C Clamp Render (Autodesk Fusion 360 archive; units mm, degrees)
design "Main Body"
part number: 2026-06-23-09-52-08-828
Autodesk Fusion 360 part; units mm, degrees
sketch "Sketch1" plane through (0, 0, 0) normal (0, 1, 0) x (1, 0, 0)
  spline S0 degree 5 poles (-77.228, -92.7344) (-75.7321, -92.7465) (-72.7402, -92.7709) (-68.2525, -92.8074) (-62.2689, -92.856) (-54.7893, -92.9168) (-48.8056, -92.9655) (-44.3179, -93.0019) (-41.3261, -93.0263) (-39.8302, -93.0384) knots 0 0 0 0 0 0 0.2 0.4 0.6 0.8 1 1 1 1 1 1
  spline S1 degree 5 poles (0, -10) (0, -14) (0, -22) (0, -34) (0, -50) (0, -70) (0, -86) (0, -98) (0, -106) (0, -110) knots 0 0 0 0 0 0 0.2 0.4 0.6 0.8 1 1 1 1 1 1
  spline S2 degree 5 poles (0, -110) (-0.2419, -110.8286) (-0.8048, -112.4078) (-1.8868, -114.5428) (-3.8082, -116.9186) (-7.0161, -119.0978) (-11.0197, -120.5038) (-15.7646, -121.2051) (-21.1395, -121.3347) (-27.004, -121.0593) (-33.2045, -120.5595) (-39.5939, -120.0074) (-46.047, -119.5474) (-52.4786, -119.2731) (-58.8364, -119.2387) (-65.0917, -119.4702) (-70.0044, -119.8743) (-73.6364, -120.2998) (-76.0347, -120.6375) (-77.228, -120.8199) knots 0 0 0 0 0 0 0.066667 0.133333 0.2 0.266667 0.333333 0.4 0.466667 0.533333 0.6 0.666667 0.733333 0.8 0.866667 0.933333 1 1 1 1 1 1
  spline S3 degree 5 poles (-39.8302, -93.0384) (-39.4353, -93.0976) (-38.6638, -93.1866) (-37.5612, -93.2318) (-36.2024, -93.1125) (-34.7008, -92.6456) (-33.4105, -91.8376) (-32.3432, -90.6698) (-31.496, -89.1468) (-30.8521, -87.2956) (-30.3924, -85.1473) (-30.158, -83.2133) (-30.0522, -81.6499) (-30.0123, -80.5582) (-30, -80) knots 0 0 0 0 0 0 0.1 0.2 0.3 0.4 0.5 0.6 0.7 0.8 0.9 1 1 1 1 1 1
  line L0 (-30, -80) -> (-30, -10)
  spline S4 degree 5 poles (-30, -10) (-30.0155, -9.1002) (-30.1233, -7.3553) (-30.5152, -4.9016) (-31.5056, -1.9629) (-33.5686, 1.1235) (-36.5062, 3.5878) (-40.343, 5.4122) (-45.0325, 6.6301) (-50.4945, 7.2984) (-56.6452, 7.4768) (-62.0611, 7.267) (-66.3821, 6.9254) (-69.376, 6.6171) (-70.9013, 6.4428) knots 0 0 0 0 0 0 0.1 0.2 0.3 0.4 0.5 0.6 0.7 0.8 0.9 1 1 1 1 1 1
  line L1 (-70.9013, 6.4428) -> (-70.9013, -3.3971)
  line L2 (-70.9013, -3.3971) -> (-100.9013, -3.3971)
  spline S5 degree 5 poles (-100.9013, -3.3971) (-100.9574, -2.1416) (-101.0166, 0.3245) (-100.9463, 3.8888) (-100.5294, 8.3669) (-99.4326, 13.476) (-97.7071, 18.0518) (-95.2994, 22.0487) (-92.1763, 25.4387) (-88.3609, 28.2411) (-83.9031, 30.4986) (-79.864, 31.9035) (-76.5855, 32.7456) (-74.2909, 33.2146) (-73.1164, 33.426) knots 0 0 0 0 0 0 0.1 0.2 0.3 0.4 0.5 0.6 0.7 0.8 0.9 1 1 1 1 1 1
  spline S6 degree 5 poles (-73.1164, 33.426) (-71.9395, 33.4424) (-69.5694, 33.474) (-65.9649, 33.5179) (-61.0595, 33.5694) (-54.7671, 33.6099) (-48.3371, 33.5898) (-41.8214, 33.4362) (-35.3156, 33.0245) (-28.9664, 32.1719) (-22.9444, 30.6684) (-17.4217, 28.305) (-12.5487, 24.9009) (-8.4236, 20.3435) (-5.087, 14.5935) (-2.547, 7.6516) (-1.1437, 1.1623) (-0.438, -4.2199) (-0.1205, -8.0354) (0, -10) knots 0 0 0 0 0 0 0.066667 0.133333 0.2 0.266667 0.333333 0.4 0.466667 0.533333 0.6 0.666667 0.733333 0.8 0.866667 0.933333 1 1 1 1 1 1
  line L3 (-77.228, -92.7344) -> (-77.228, -120.8199)
  line L4 (-77.228, -120.8199) -> (-107.228, -120.8199)
  line L5 (-107.228, -120.8199) -> (-107.228, -92.3319)
  line L6 (-107.228, -92.3319) -> (-77.228, -92.3319)
  line L7 (-77.228, -92.3319) -> (-77.228, -120.8199)
  point P0 (-10, -120)
  point P1 (-40, -120)
  point P2 (-32.9581, -91.2668)
  point P3 (-36.8896, 3.5278)
  point P4 (-94.8799, 22.2135)
  point P5 (-43.1491, 33.426)
  point P6 (-14.9821, 26.4017)
  dimension "d1" = 30
  dimension "d4" = 30
  constraint vertical L0
  constraint vertical L1
  constraint perpendicular L1 L2
  constraint vertical L3
  constraint horizontal L4
  constraint vertical L5
  constraint horizontal L6
  constraint vertical L7
  measures "d1" distance of L1.end L2.end
  measures "d4" distance of S2.end L4.end
sketch "Sketch2" plane through (0, 0, 0) normal (0, 1, 0) x (1, 0, 0)
extrude "Extrude2" add sketch "Sketch1" along normal blind 10 contours S0 S1 S2 S3 L0 S4 L1 L2 S5 S6 L3 L7 makes body 1
sketch "Sketch3" plane through (0, 0, 0) normal (0, 0, 1) x (1, 0, 0)
  circle A0 centre (40, 0) radius 10
  dimension "d7" = 20
  measures "d7" diameter of A0
extrude "Extrude3" add sketch "Sketch3" along normal blind 30 separate body makes body 2
move_body "Move1" bodies 2 to x (0.642788, 0.766044, 0) y (-0.766044, 0.642788, 0) z (0, 0, 1) at (-113.2291, -9.4059, 86.4551)
move_body "Move2" bodies 2 to x (1, 0, 0) y (0, 1, 0) z (0, 0, 1) at (0, -16, 6)
sketch "Sketch4" plane through (0, 0, 122.4551) normal (0, 0, 1) x (-1, 0, 0)
  circle A0 centre (87.5176, -5.2359) radius 10
  circle A1 centre (87.5176, -5.2359) radius 3
  dimension "d12" = 6
  constraint concentric A0 A1
  measures "d12" diameter of A1
extrude "Extrude4" cut sketch "Sketch4" against normal blind 57 contours A1 bodies 2
extrude "Extrude1" [suppressed]
